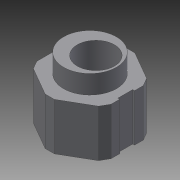
# Autodesk Inventor part: OpenBuilds_Eccentric_Spacer
Saved by Autodesk Inventor 2014 (Build 180170000, 170)
## iProperties
Created: 2014-08-25
Part Number: OpenBuilds_Eccentric_Spacer
Material: Generic
Document SubType Name: Modeling
Designer: ThatOtherGuy
Density: 1 g/cm^3
Appearance: Default
Author: ThatOtherGuy
Autodesk Inventor part; units mm, degrees
ref_plane "YZ Plane" through (0, 0, 0) normal (1, 0, 0) x (0, 1, 0)
ref_plane "XZ Plane" through (0, 0, 0) normal (0, 1, 0) x (-1, 0, 0)
ref_plane "XY Plane" through (0, 0, 0) normal (0, 0, 1) x (1, 0, 0)
sketch "Sketch1" plane through (0, 0, 0) normal (0, 0, 1) x (1, 0, 0)
  circle A0 centre (0, 0) radius 3.555
  line L0 (0, 5.7735) -> (5, 2.8868)
  line L1 (5, 2.8868) -> (5, -2.8868)
  line L2 (5, -2.8868) -> (0, -5.7735)
  line L3 (0, -5.7735) -> (-5, -2.8868)
  line L4 (-5, -2.8868) -> (-5, 2.8868)
  line L5 (-5, 2.8868) -> (0, 5.7735)
  circle A1 centre (0.79, 0) radius 2.5
  dimension "d0" = 7.11
  dimension "d2" = 10
  dimension "d3" = 5
  dimension "d4" = 0.79
  constraints: 12 end point, 2 centre point, 2 coincident, 1 horizontal alignment, 1 vertical, 13 other
  measures "d0" diameter of A0
  measures "d2" distance between parallel lines of L2 L5
  measures "d3" diameter of A1
  measures "d4" distance of point (0, 0) A1.centre
extrude "Extrusion1" add sketch "Sketch1" along normal blind 6.35 contours A0 | L0 L1 L2 L3 L4 L5
sketch "Sketch2" plane through (0, 0, 6.35) normal (0, 0, 1) x (1, 0, 0)
  circle A0 centre (0.79, 0) radius 2.5 projected
  circle A1 centre (0, 0) radius 3.555
  circle A2 centre (0.79, 0) radius 2.5
  dimension "d7" = 7.11
  dimension "d9" = 5
  constraints: 4 coincident, 2 centre point, 1 horizontal alignment
  measures "d7" diameter of A1
  measures "d9" diameter of A2
extrude "Extrusion2" add sketch "Sketch2" along normal blind 2.5
sketch "Sketch3" plane through (5, -2.8868, 0) normal (1, 0, 0) x (0, 0, -1)
  line L0 (0, 5.7735) -> (0, 0) projected
  line L1 (-6.35, 0) -> (-6.35, 5.7735) projected
  line L2 (-6.35, 3.8868) -> (0, 3.8868)
  line L3 (0, 1.8868) -> (-6.35, 1.8868)
  line L4 (-6.35, 2.8868) -> (0, 2.8868) construction
  line L5 (-1.966, 2.8868) -> (-1.966, 3.8868) construction
  line L6 (-1.966, 2.8868) -> (-1.966, 1.8868) construction
  dimension "d13" = 2
  constraints: 10 end point, 7 point on line, 3 perpendicular, 2 equal length, 1 collinear, 1 midpoint
  measures "d13" distance between parallel lines of L3 L2
extrude "Extrusion3" cut sketch "Sketch3" against normal blind 0.25
sketch "Sketch4" plane through (0, 0, 6.35) normal (0, 0, 1) x (1, 0, 0)
  line L0 (3.1264, 5.415) -> (6.2527, 0)
  line L1 (6.2527, 0) -> (3.1264, -5.415)
  line L2 (3.1264, -5.415) -> (-3.1264, -5.415)
  line L3 (-3.1264, -5.415) -> (-6.2527, 0)
  line L4 (-6.2527, 0) -> (-3.1264, 5.415)
  line L5 (-3.1264, 5.415) -> (3.1264, 5.415)
  line L6 (-3.1264, 5.415) -> (0, 7.4304)
  line L7 (0, 7.4304) -> (3.1264, 5.415)
  line L8 (-3.1264, 5.415) -> (-7.0189, 5.2081)
  line L9 (-7.0189, 5.2081) -> (-6.2527, 0)
  line L10 (-6.2527, 0) -> (-7.6169, -4.7381)
  line L11 (-7.6169, -4.7381) -> (-3.1264, -5.415)
  line L12 (-3.1264, -5.415) -> (-0.7756, -8.4436)
  line L13 (-0.7756, -8.4436) -> (3.1264, -5.415)
  line L14 (3.1264, -5.415) -> (7.3563, -3.9182)
  line L15 (7.3563, -3.9182) -> (6.2527, 0)
  line L16 (6.2527, 0) -> (7.7493, 2.746)
  line L17 (7.7493, 2.746) -> (3.1264, 5.415)
  point P0 (0, 0)
  point P1 (0, 0)
  dimension "d16" = 10.83
  constraints: 36 end point, 2 perpendicular, 1 coincident, 1 horizontal, 13 other
  measures "d16" distance between parallel lines of L2 L5
extrude "Extrusion4" cut sketch "Sketch4" against normal up to surface (6.35 mm away) contours L17 L16 L0 | L5 L6 L7 | L15 L14 L1 | L4 L9 L8 | L13 L12 L2 | L3 L11 L10
body "Solid1"
